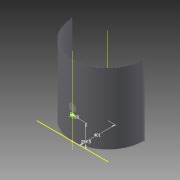
# Autodesk Inventor part: Lower Back Half
Saved by Autodesk Inventor 2015 (Build 190159000, 159)
## iProperties
Created: 2014-06-19
Part Number: Lower Back Half
Material: Generic
Document SubType Name: Modeling
Designer: Aki
Density: 1 g/cm^3
Appearance: Default
Author: Aki
Autodesk Inventor part; units mm, degrees
ref_plane "YZ Plane" through (0, 0, 0) normal (1, 0, 0) x (0, 1, 0)
ref_plane "XZ Plane" through (0, 0, 0) normal (0, 1, 0) x (-1, 0, 0)
ref_plane "XY Plane" through (0, 0, 0) normal (0, 0, 1) x (1, 0, 0)
sketch "Sketch1" plane through (0, 0, 0) normal (0, 1, 0) x (-1, 0, 0)
  arc A0 (401, 0) -> (-401, 0) centre (0, 0) ccw
  line L0 (0, 0) -> (-401, 0) construction
  line L1 (0, 0) -> (401, 0) construction
  arc A1 (400, 0) -> (-400, 0) centre (0, 0) ccw
  line L2 (0, 0) -> (-400, 0) construction
  line L3 (0, 0) -> (400, 0) construction
  line L4 (-401, 0) -> (-400, 0)
  line L5 (400, 0) -> (401, 0)
  dimension "d0" = 401
  dimension "d1" = 180
  dimension "d2" = 400
  dimension "d3" = 180
  constraints: 12 end point, 4 point on circle, 2 centre point, 2 coincident, 1 collinear
  measures "d0" radius of A0
  measures "d1" angle of L0 L1
  measures "d2" radius of A1
  measures "d3" angle of L2 L3
extrude "Extrusion1" add sketch "Sketch1" along normal blind 796
sketch "Sketch2" plane through (0, 0, 0) normal (0, 1, 0) x (-1, 0, 0)
  line L0 (-401, 0) -> (-416, 0)
  line L1 (-416, 0) -> (-416, 1)
  line L2 (-416, 1) -> (-401, 1)
  line L3 (-401, 1) -> (-401, 0)
  point P0 (0, 0)
  dimension "d6" = 15
  dimension "d7" = 1
  constraints: 8 end point, 2 parallel, 1 horizontal, 1 perpendicular
  measures "d6" distance of L1.end L2.end
  measures "d7" distance of L0.end L1.end
extrude "Extrusion2" add sketch "Sketch2" along normal blind 796
sketch "Sketch3" plane through (0, 0, 0) normal (0, 1, 0) x (-1, 0, 0)
  line L0 (401, 0) -> (416, 0)
  line L1 (416, 0) -> (416, 1)
  line L2 (416, 1) -> (401, 1)
  line L3 (401, 1) -> (401, 0)
  point P0 (0, 0)
  dimension "d10" = 15
  dimension "d11" = 1
  constraints: 8 end point, 2 parallel, 1 horizontal, 1 perpendicular
  measures "d10" distance of L2.end L1.end
  measures "d11" distance of L1.end L0.end
extrude "Extrusion3" add sketch "Sketch3" along normal blind 796
sketch "Sketch4" plane through (0, 0, 0) normal (0, 1, 0) x (-1, 0, 0)
  line L0 (0, 0) -> (0, 401)
  dimension "d14" = 401
  constraints: 2 end point, 1 vertical
  measures "d14" distance of L0.start L0.end
ref_plane "Work Plane1" through (0, 0, 401) normal (0, 0, 1) x (1, 0, 0)
sketch "Sketch5" plane through (0, 0, 401) normal (0, 0, 1) x (1, 0, 0)
  circle A0 centre (0, 254.5) radius 25
  line L0 (401, 0) -> (-401, 0) projected
  point P0 (0, 0)
  dimension "d15" = 50
  dimension "d16" = 254.5
  constraints: 1 centre point
  measures "d15" diameter of A0
  measures "d16" distance from line of L0 A0.centre
hole "Hole1" at (0, 254.5, 401) direction (0, 0, -1) diameter 50 end through all
sketch "Sketch6" plane through (0, 0, 401) normal (0, 0, 1) x (1, 0, 0)
  circle A0 centre (0, 330.5) radius 42
  line L0 (401, 0) -> (-401, 0) projected
  point P0 (0, 0)
  dimension "d24" = 84
  dimension "d25" = 330.5
  constraints: 1 centre point
  measures "d24" diameter of A0
  measures "d25" distance from line of L0 A0.centre
hole "Hole2" at (0, 330.5, 401) direction (0, 0, -1) diameter 84 end through all
sketch "Sketch7" plane through (0, 0, 401) normal (0, 0, 1) x (1, 0, 0)
  circle A0 centre (0, 254.5) radius 25
  line L0 (401, 0) -> (-401, 0) projected
  point P0 (0, 0)
  dimension "d33" = 50
  dimension "d34" = 254.5
  constraints: 1 centre point
  measures "d33" diameter of A0
  measures "d34" distance from line of L0 A0.centre
body "Solid1"
